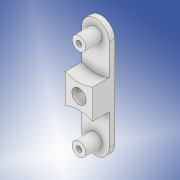
# Autodesk Inventor part: WaveGenerator
Saved by Autodesk Inventor 2017 (Build 210142000, 142)
## iProperties
Created: 2017-07-11
Part Number: WaveGenerator
Material: ABS Plastic
Document SubType Name: Modeling
Designer: zallen
Density: 1.06 g/cm^3
Appearance: CR White
Author: zallen
Autodesk Inventor part; units mm, degrees
ref_plane "YZ Plane" through (0, 0, 0) normal (1, 0, 0) x (0, 1, 0)
ref_plane "XZ Plane" through (0, 0, 0) normal (0, 1, 0) x (-1, 0, 0)
ref_plane "XY Plane" through (0, 0, 0) normal (0, 0, 1) x (1, 0, 0)
sketch "Sketch1" plane through (0, 0, 0) normal (0, 0, 1) x (1, 0, 0)
  line L0 (0, 0) -> (0, 65) construction
  circle A0 centre (0, 57.5) radius 7.5 construction
  circle A1 centre (0, 7.5) radius 7.5 construction
  line L1 (7.5, 57.5) -> (7.5, 7.5)
  line L2 (-7.5, 7.5) -> (-7.5, 57.5)
  arc A2 (7.5, 57.5) -> (-7.5, 57.5) centre (0, 57.5) ccw
  arc A3 (-7.5, 7.5) -> (7.5, 7.5) centre (0, 7.5) ccw
  circle A4 centre (0, 32.5) radius 3.9
  circle A5 centre (0, 57.5) radius 3.75
  circle A6 centre (0, 7.5) radius 3.75
  dimension "d0" = 65
  dimension "d1" = 15
  dimension "d2" = 15
  dimension "d3" = 7.8
  dimension "d4" = 7.5
  dimension "d5" = 7.5
  constraints: 10 point on circle, 7 centre point, 6 end point, 6 tangent, 2 coincident, 2 point on line, 1 concentric, 1 midpoint, 1 vertical
  measures "d0" distance of L0.start L0.end
  measures "d1" diameter of A0
  measures "d2" diameter of A1
  measures "d3" diameter of A4
  measures "d4" diameter of A5
  measures "d5" diameter of A6
extrude "Extrusion1" add sketch "Sketch1" along normal blind 3
sketch "Sketch3" plane through (0, 0, 0) normal (0, 0, -1) x (-1, 0, 0)
  circle A0 centre (0, 57.5) radius 3.75 projected
  circle A1 centre (0, 7.5) radius 3.75 projected
  point P0 (0, 0)
extrude "Extrusion2" add sketch "Sketch3" against normal blind 12
sketch "Sketch4" plane through (0, 57.5, 12) normal (0, 0, 1) x (1, 0, 0)
  circle A0 centre (0, 0) radius 3.75 projected
  circle A1 centre (0, -50) radius 3.75 projected
  circle A2 centre (0, 0) radius 1.5
  circle A3 centre (0, -50) radius 1.5
  point P0 (0, -57.5)
  dimension "d10" = 3
  dimension "d11" = 3
  constraints: 2 centre point, 2 coincident
  measures "d10" diameter of A2
  measures "d11" diameter of A3
extrude "Extrusion3" cut sketch "Sketch4" against normal through all contours A2 | A3
sketch "Sketch5" plane through (0, 0, 3) normal (0, 0, 1) x (1, 0, 0)
  arc A0 (7.5, 57.5) -> (-7.5, 57.5) centre (0, 57.5) ccw projected
  arc A1 (-7.5, 7.5) -> (7.5, 7.5) centre (0, 7.5) ccw projected
  circle A2 centre (0, 57.5) radius 1.5 projected
  circle A3 centre (0, 57.5) radius 18.5 construction
  circle A4 centre (0, 7.5) radius 18.5 construction
  line L0 (7.5, 7.5) -> (7.5, 57.5) projected
  line L1 (7.5, 40.5885) -> (7.5, 24.4115)
  line L2 (-7.5, 57.5) -> (-7.5, 7.5) projected
  line L3 (-7.5, 40.5885) -> (-7.5, 24.4115)
  arc A5 (-7.5, 40.5885) -> (7.5, 40.5885) centre (0, 57.5) ccw
  arc A6 (7.5, 24.4115) -> (-7.5, 24.4115) centre (0, 7.5) ccw
  circle A7 centre (0, 32.5) radius 3.9 projected
  point P0 (0, 0)
  dimension "d14" = 37
  dimension "d15" = 37
  constraints: 8 point on circle, 4 centre point, 4 end point, 4 point on line, 2 coincident, 2 concentric
  measures "d14" diameter of A3
  measures "d15" diameter of A4
extrude "Extrusion4" add sketch "Sketch5" along normal blind 9 contours L0 A6 L2 A5
sketch "Sketch6" plane through (0, 0, 0) normal (1, 0, 0) x (0, 1, 0)
  line L0 (7.5, 0) -> (57.5, 0) projected
  line L1 (7.5, 0) -> (7.5, 3) projected
  line L2 (24.4115, 3) -> (7.5, 3) projected
  line L3 (24.4115, 3) -> (24.4115, 12) projected
  line L4 (40.5885, 12) -> (24.4115, 12) projected
  line L5 (40.5885, 3) -> (40.5885, 12) projected
  line L6 (57.5, 3) -> (40.5885, 3) projected
  line L7 (57.5, 0) -> (57.5, 3) projected
  circle A0 centre (32.5, 7.5) radius 1.5
  point P0 (0, 0)
  point P1 (32.5, 12)
  point P2 (40.5885, 7.5)
  dimension "d18" = 3
  constraints: 2 midpoint, 1 centre point, 1 horizontal alignment, 1 vertical alignment
  measures "d18" diameter of A0
extrude "Extrusion5" cut sketch "Sketch6" against normal through all contours A0
body "Solid1"
